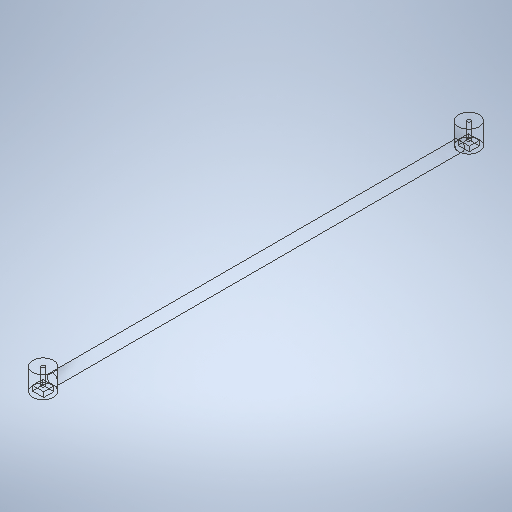
# Autodesk Inventor part: Solar_Panel_Bar
Saved by Autodesk Inventor 2025 (Build 290162010, 162A)
## iProperties
Created: 2024-07-15
Part Number: Solar_Panel_Bar
Material: Generic
Document SubType Name: Modeling
Designer: vncnt
Density: 1 g/cm^3
Appearance: Default
Author: vncnt
Autodesk Inventor part; units mm, degrees
ref_plane "YZ Plane" through (0, 0, 0) normal (1, 0, 0) x (0, 1, 0)
ref_plane "XZ Plane" through (0, 0, 0) normal (0, 1, 0) x (-1, 0, 0)
ref_plane "XY Plane" through (0, 0, 0) normal (0, 0, 1) x (1, 0, 0)
sketch "Sketch1" plane through (0, 0, 0) normal (0, 0, 1) x (1, 0, 0)
  circle A0 centre (0, 0) radius 3.175
  dimension "d0" = 6.35
  constraints: 1 centre point, 1 coincident
  measures "d0" diameter of A0
extrude "Extrusion1" add sketch "Sketch1" along normal mid plane 259
sketch "Sketch2" plane through (0, 0, 0) normal (0, 1, 0) x (-1, 0, 0)
  circle A0 centre (0, 129.875) radius 6.35
  circle A1 centre (0, -129.875) radius 6.35
  line L0 (-3.175, -129.5) -> (-3.175, 129.5) projected
  line L1 (-3.175, 0) -> (16.7407, 0)
  point P0 (3.175, -105.625)
  dimension "d4" = 259.75
  dimension "d5" = 129.875
  dimension "d6" = 12.7
  dimension "d7" = 12.7
  constraints: 2 centre point, 2 end point, 1 horizontal, 1 midpoint
  measures "d4" distance of A0.centre A1.centre
  measures "d5" distance from line of L1 A0.centre
  measures "d6" diameter of A0
  measures "d7" diameter of A1
extrude "Extrusion2" add sketch "Sketch2" along normal blind 10 and the other way blind 3.175
sketch "Sketch3" plane through (0, 10, 129.875) normal (0, 1, 0) x (1, 0, 0)
  circle A0 centre (0, 0) radius 6.35 projected
  circle A1 centre (0, 259.75) radius 6.35 projected
  point P0 (0, 129.875)
  constraints: 2 coincident
hole "Hole1" at (0, 10, 129.875) at (0, 10, -129.875) direction (0, -1, 0) diameter 2.1565 end through all thread size "4-40 UNC" class "2B" standard "ANSI Unified Screw Threads"
sketch "Sketch9" plane through (0, -3.175, 129.875) normal (0, -1, 0) x (1, 0, 0)
  line L0 (-3.45, 3.1) -> (3.45, 3.1)
  line L1 (3.45, 3.1) -> (3.45, -3.1)
  line L2 (3.45, -3.1) -> (-3.45, -3.1)
  line L3 (-3.45, -3.1) -> (-3.45, 3.1)
  line L4 (-3.45, 3.1) -> (3.45, -3.1) construction
  line L5 (3.45, 3.1) -> (-3.45, -3.1) construction
  line L6 (0, -129.875) -> (-12.946, -129.875)
  line L7 (-3.45, -262.85) -> (3.45, -262.85)
  line L8 (3.45, -262.85) -> (3.45, -256.65)
  line L9 (3.45, -256.65) -> (-3.45, -256.65)
  line L10 (-3.45, -256.65) -> (-3.45, -262.85)
  point P0 (0, 0)
  dimension "d28" = 6.9
  dimension "d29" = 6.2
  constraints: 22 end point, 4 symmetric about line, 2 horizontal, 2 midpoint, 2 parallel, 1 perpendicular
  measures "d28" distance of L1.end L2.end
  measures "d29" distance of L0.end L1.end
extrude "Extrusion6" cut sketch "Sketch9" against normal blind 3
body "Solid1"
